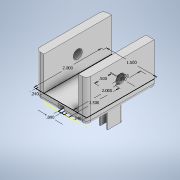
# Autodesk Inventor part: Sample Holder Clip for Plates-v2
Saved by Autodesk Inventor 2020 (Build 240168000, 168)
## iProperties
Created: 2022-02-13
Part Number: Sample Holder Clip for Plates-v2
Material: Generic
Document SubType Name: Modeling
Designer: Beaucage
Density: 1 g/cm^3
Appearance: Default
Author: Beaucage
Autodesk Inventor part; units mm, degrees
ref_plane "YZ Plane" through (0, 0, 0) normal (1, 0, 0) x (0, 1, 0)
ref_plane "XZ Plane" through (0, 0, 0) normal (0, 1, 0) x (-1, 0, 0)
ref_plane "XY Plane" through (0, 0, 0) normal (0, 0, 1) x (1, 0, 0)
sketch "Sketch1" plane through (0, 0, 0) normal (0, 1, 0) x (-1, 0, 0)
  line L0 (0, 0) -> (38.1, 0)
  line L1 (38.1, 0) -> (38.1, -50.8)
  line L2 (38.1, -50.8) -> (0, -50.8)
  line L3 (0, -50.8) -> (0, 0)
  line L4 (38.1, -50.8) -> (32.004, -50.8)
  line L5 (32.004, -50.8) -> (32.004, 0)
  line L6 (32.004, 0) -> (38.1, 0)
  line L7 (38.1, 0) -> (38.1, -50.8)
  line L8 (0, -50.8) -> (6.096, -50.8)
  line L9 (6.096, -50.8) -> (6.096, 0)
  line L10 (6.096, 0) -> (0, 0)
  line L11 (0, 0) -> (0, -50.8)
  dimension "d0" = 38.1
  dimension "d1" = 50.8
  dimension "d2" = 6.096
  dimension "d3" = 6.096
  dimension "d4" = 50.8
  constraints: 24 end point, 6 parallel, 3 horizontal, 3 perpendicular, 1 point on line
  measures "d0" distance of L1.end L2.end
  measures "d1" distance of L0.end L1.end
  measures "d2" distance of L5.end L6.end
  measures "d3" distance of L10.end L9.end
  measures "d4" distance of L9.end L8.end
extrude "Extrusion1" add sketch "Sketch1" along normal blind 25.4 contours L0 L9 L2 L3 | L0 L1 L2 L5
extrude "Extrusion2" add sketch "Sketch1" against normal blind 6.35
sketch "Sketch2" plane through (0, -6.35, 0) normal (0, -1, 0) x (1, 0, 0)
  line L0 (-32.004, 0) -> (-6.096, 0) projected
  line L1 (-19.05, 0) -> (-16.764, 0)
  line L2 (-16.764, 0) -> (-16.764, -38.1)
  line L3 (-16.764, -38.1) -> (-19.05, -38.1)
  line L4 (-19.05, -38.1) -> (-19.05, 0)
  line L5 (-19.05, -38.1) -> (-21.336, -38.1)
  line L6 (-21.336, -38.1) -> (-21.336, 0)
  line L7 (-21.336, 0) -> (-19.05, 0)
  line L8 (-19.05, 0) -> (-19.05, -38.1)
  line L9 (-15.875, -31.75) -> (-22.225, -31.75)
  line L10 (-22.225, -31.75) -> (-22.225, -44.45)
  line L11 (-22.225, -44.45) -> (-15.875, -44.45)
  line L12 (-15.875, -44.45) -> (-15.875, -31.75)
  line L13 (-15.875, -31.75) -> (-22.225, -44.45) construction
  line L14 (-22.225, -31.75) -> (-15.875, -44.45) construction
  point P0 (0, 0)
  point P1 (-16.764, 0)
  point P2 (-21.336, 0)
  point P3 (-16.764, -31.75)
  point P4 (-21.336, -31.75)
  dimension "d9" = 2.286
  dimension "d10" = 38.1
  dimension "d11" = 2.286
  dimension "d12" = 6.35
  dimension "d13" = 12.7
  constraints: 28 end point, 6 parallel, 3 horizontal, 3 midpoint, 3 perpendicular, 1 point on line
  measures "d9" distance of L2.end L3.end
  measures "d10" distance of L1.end L2.end
  measures "d11" distance of L6.end L7.end
  measures "d12" distance of L11.end L10.end
  measures "d13" distance of L10.end L9.end
extrude "Extrusion3" cut sketch "Sketch2" against normal blind 5.08 contours L0 L4 L9 L6 | L0 L2 L9 L4 | L9 L4 L5 L6 | L9 L2 L3 L4
extrude "Extrusion4" add sketch "Sketch2" along normal blind 25.4 contours L6 L5 L3 L2 L9 L12 L11 L10
fillet "Fillet1" radius 3.175 9 edges at (0, -6.35, -25.4) (0, 9.525, 0) (-15.875, -19.05, -44.45) (-8.382, -6.35, 0) (-29.718, -6.35, 0) (-19.05, -6.35, -50.8) (-38.1, -6.35, -25.4) (-22.225, -19.05, -44.45) (-19.05, -31.75, -44.45)
fillet "Fillet2" radius 3.175 7 edges at (-19.05, -6.35, -44.45) (-15.875, -6.35, -36.5125) (-22.225, -6.35, -36.5125) (-37.1701, -5.4201, -0.9299) (-38.1, 11.1125, 0) (-37.1701, -5.4201, -49.8701) (-38.1, 11.1125, -50.8)
sketch "Sketch3" plane through (-38.1, -3.175, -47.625) normal (-1, 0, 0) x (0, 0, 1)
  line L0 (47.625, 3.175) -> (-3.175, 3.175) projected
  line L1 (-3.175, 3.175) -> (47.625, 3.175) projected
  line L2 (22.225, 3.175) -> (22.225, 15.875)
  dimension "d20" = 12.7
  constraints: 2 end point, 1 midpoint, 1 vertical
  measures "d20" distance of L2.start L2.end
hole "Hole1" at (-38.1, 12.7, -25.4) direction (1, 0, 0) diameter 6.7564 end through all clearance for "Flat Head Machine Screw (82)" size "1/4" standard "Ansi Unified Screw Threads"
body "Solid1"
